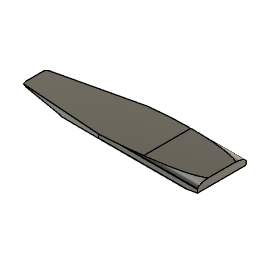
body v3 (Autodesk Fusion 360 design; units mm, degrees)
Autodesk Fusion 360 part; units mm, degrees
sketch "Sketch1" plane through (0, 0, 0) normal (0, 1, 0) x (1, 0, 0)
  line L0 (0, 0) -> (3657.6, 0) construction
  line L1 (0, -9.144) -> (2590.8, -201.168)
  line L2 (2590.8, -201.168) -> (3651.504, -259.08)
  line L3 (3651.504, -259.08) -> (3651.504, -105.156)
  line L4 (3651.504, -105.156) -> (2464.308, 126.492)
  line L5 (0, -9.144) -> (0, 3.048)
  line L6 (0, 3.048) -> (829.056, 36.576)
  line L7 (829.056, 36.576) -> (1645.92, 152.4)
  line L8 (1645.92, 152.4) -> (2464.308, 126.492)
  dimension "d1" = 3657.6
  constraint coincident L0.start origin
  constraint horizontal L0
  constraint perpendicular L0 L3
  constraint perpendicular L0 L5
  measures "d1" distance of L0.start L0.end
extrude "Extrude1" add sketch "Sketch1" along normal blind 950.976
sketch "Sketch3" plane through (0, 0, 0) normal (0, 0, 1) x (1, 0, 0)
  line L0 (3657.6, 0) -> (3657.6, 950.976)
  dimension "d4" = 950.976
  constraint vertical L0
  measures "d4" distance of L0.start L0.end
ref_plane "WorkPlane1" through (0, 0, 609.6) normal (0, 0, 1) x (1, 0, 0)
sketch "Sketch5" plane through (0, 0, 609.6) normal (0, 0, 1) x (1, 0, 0)
sketch "Sketch4" plane through (0, 0, 609.6) normal (0, 0, 1) x (1, 0, 0)
  line L0 (0, 0) -> (0, 950.976)
  line L1 (0, 475.488) -> (3657.5999, 475.488)
  line L2 (1755.648, 950.976) -> (59.327, 713.8559)
  line L3 (50.5889, 711.807) -> (37.6015, 707.4778)
  line L4 (9.1835, 682.8311) -> (0, 664.464)
  line L5 (0, 950.976) -> (1755.648, 950.976)
  arc A0 (37.6015, 707.4778) -> (9.1835, 682.8311) centre (53.1437, 660.851) ccw
  arc A1 (59.327, 713.8559) -> (50.5889, 711.807) centre (66.1311, 665.1801) ccw
  line L6 (1755.648, 0) -> (59.327, 237.1201)
  arc A2 (50.5889, 239.169) -> (59.327, 237.1201) centre (66.1311, 285.7959) ccw
  line L7 (50.5889, 239.169) -> (37.6015, 243.4982)
  arc A3 (9.1835, 268.1449) -> (37.6015, 243.4982) centre (53.1437, 290.125) ccw
  line L8 (9.1835, 268.1449) -> (0, 286.512)
  line L9 (0, 0) -> (1755.648, 0)
  dimension "d5" = 49.149
  constraint coincident L0.start L9.start
  constraint vertical L0
  constraint midpoint L0 L1.start
  constraint perpendicular L0 L1
  constraint coincident L0 L4.end
  constraint perpendicular L0 L5
  constraint tangent L4 A0
  constraint tangent L3 A0
  constraint tangent L3 A1
  constraint tangent L2 A1
  constraint equal A0 A1
  constraint symmetric L0.end L1 L0.start
  constraint symmetric L1 L2.start L6.start
  constraint symmetric L1 L4.end L8.end
  constraint symmetric L1 L4.start A3.start
  constraint symmetric L1 L3.end L7.end
  constraint symmetric L1 A0 A3
  constraint symmetric L1 L3.start A2.start
  constraint symmetric L1 L2.end L6.end
  constraint symmetric L1 A1 A2
  measures "d5" radius of A0
extrude "Extrude3" cut sketch "Sketch4" against normal blind 1005.84
sketch "Sketch6" plane through (0, 0, 0) normal (1, 0, 0) x (0, 1, 0)
  line L0 (975.36, 274.32) -> (-30.48, 274.32)
  line L1 (-30.48, 274.32) -> (-30.48, -182.88)
  line L2 (-30.48, -182.88) -> (975.36, -182.88)
  line L3 (975.36, -182.88) -> (975.36, 274.32)
  line L4 (950.976, 259.08) -> (0, 259.08) construction
  line L5 (475.488, 259.08) -> (475.488, 329.184)
  line L6 (475.488, 329.184) -> (475.488, -259.9361)
  line L7 (475.488, 259.08) -> (743.712, 259.08)
  line L8 (950.6039, 169.7136) -> (945.1676, 66.4238)
  line L9 (940.9107, 57.1943) -> (737.6274, -135.6643)
  line L10 (707.136, -164.592) -> (707.136, -182.88)
  spline S0 degree 5 poles (743.712, 259.08) (746.3796, 258.8054) (751.6686, 258.2475) (759.4637, 257.3843) (769.5788, 256.1803) (781.7643, 254.5815) (793.5174, 252.8745) (804.9017, 251.0321) (816.0295, 249.0107) (827.0873, 246.7445) (838.3149, 244.1487) (849.9297, 241.1323) (862.0647, 237.6086) (874.7007, 233.5076) (887.597, 228.788) (900.2199, 223.4503) (911.9081, 217.5377) (922.0259, 211.1385) (930.136, 204.3899) (936.1341, 197.479) (940.4921, 190.6573) (943.39, 185.4946) (945.6182, 181.8896) (947.1853, 179.6184) (947.9893, 178.5158) knots 0 0 0 0 0 0 0.05 0.1 0.15 0.2 0.25 0.3 0.35 0.4 0.45 0.5 0.55 0.6 0.65 0.7 0.75 0.8 0.85 0.9 0.95 1 1 1 1 1 1
  arc A0 (950.6039, 169.7136) -> (947.9893, 178.5158) centre (936.9068, 170.4345) ccw
  arc A1 (940.9107, 57.1943) -> (945.1676, 66.4238) centre (931.4705, 67.1447) ccw
  line L11 (475.488, -152.4) -> (695.671, -152.4)
  arc A2 (695.671, -152.4) -> (737.6274, -135.6643) centre (695.671, -91.44) ccw
  line L12 (0, 259.08) -> (950.976, 259.08) construction
  spline S1 degree 5 poles (207.264, 259.08) (204.5964, 258.8054) (199.3074, 258.2475) (191.5124, 257.3843) (181.3972, 256.1803) (169.2117, 254.5815) (157.4586, 252.8745) (146.0743, 251.0321) (134.9465, 249.0107) (123.8887, 246.7445) (112.6611, 244.1487) (101.0464, 241.1323) (88.9113, 237.6086) (76.2753, 233.5076) (63.379, 228.788) (50.7561, 223.4503) (39.0679, 217.5377) (28.9501, 211.1385) (20.84, 204.3899) (14.8419, 197.479) (10.4839, 190.6573) (7.586, 185.4946) (5.3579, 181.8896) (3.7907, 179.6184) (2.9867, 178.5158) knots 0 0 0 0 0 0 0.05 0.1 0.15 0.2 0.25 0.3 0.35 0.4 0.45 0.5 0.55 0.6 0.65 0.7 0.75 0.8 0.85 0.9 0.95 1 1 1 1 1 1
  line L13 (717.3108, 261.7973) -> (770.1132, 256.3627)
  line L14 (935.3956, 195.7866) -> (960.5831, 161.245)
  line L15 (233.6652, 261.7973) -> (180.8628, 256.3627)
  line L16 (15.5804, 195.7866) -> (-9.6071, 161.245)
  line L17 (0.3721, 169.7136) -> (5.8084, 66.4238)
  arc A3 (2.9867, 178.5158) -> (0.3721, 169.7136) centre (14.0692, 170.4345) ccw
  arc A4 (5.8084, 66.4238) -> (10.0653, 57.1943) centre (19.5055, 67.1447) ccw
  line L18 (10.0653, 57.1943) -> (213.3486, -135.6643)
  arc A5 (213.3486, -135.6643) -> (255.305, -152.4) centre (255.305, -91.44) ccw
  line L19 (475.488, -152.4) -> (255.305, -152.4)
  line L20 (207.264, 259.08) -> (475.488, 259.08)
  point P0 (810.768, 249.936)
  point P1 (874.5914, 233.4128)
  point P2 (932.688, 201.168)
  point P3 (140.208, 249.936)
  point P4 (76.3846, 233.4128)
  point P5 (18.288, 201.168)
  dimension "d13" = 13.716
  dimension "d14" = 60.96
  constraint horizontal L0
  constraint vertical L1
  constraint horizontal L2
  constraint vertical L3
  constraint perpendicular L1 L4
  constraint midpoint L4 L5.start
  constraint perpendicular L0 L5
  constraint perpendicular L2 L6
  constraint coincident L4 L7.end
  constraint perpendicular L6 L7
  constraint coincident L2 L10.end
  constraint perpendicular L2 L10
  constraint tangent S0 A0
  constraint tangent L8 A0
  constraint tangent L8 A1
  constraint tangent L9 A1
  constraint equal A0 A1
  constraint coincident L6 L11.start
  constraint perpendicular L6 L11
  constraint coincident L10.start L9
  constraint tangent L9 A2
  constraint tangent L11 A2
  constraint midpoint L7.end L13
  constraint midpoint S0.end L14
  constraint symmetric L4.start L6 L4.end
  constraint symmetric L4.end L6 L4.start
  constraint symmetric L6 L7.end S1.start
  constraint symmetric L6 P0 P3
  constraint symmetric L6 P1 P4
  constraint symmetric L6 P2 P5
  constraint symmetric L6 S0.end S1.end
  constraint symmetric L6 A0 A3
  constraint symmetric L6 L8.start L17.start
  constraint symmetric L6 L8.end L17.end
  constraint symmetric L6 L9.start A4.end
  constraint symmetric L6 A1 A4
  constraint symmetric L6 L11.start L19.start
  constraint symmetric L6 L9.end L18.end
  constraint symmetric L6 L11.end A5.end
  constraint symmetric L6 A2 A5
  constraint symmetric L6 L13.start L15.start
  constraint symmetric L6 L13.end L15.end
  constraint symmetric L6 L14.start L16.start
  constraint symmetric L6 L14.end L16.end
  measures "d13" radius of A0
  measures "d14" radius of A2
extrude "Extrude4" cut sketch "Sketch6" along normal blind 3962.4 contours L0 L2 L3 L5 L6 L7 L8 L9 S0 A0 A1 L11 A2 | L0 L1 L2 L5 L6 S1 L17 A3 A4 L18 A5 L19 L20
